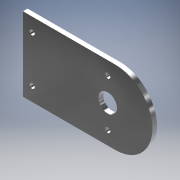
# Autodesk Inventor part: Motor Plate
Saved by Autodesk Inventor 2019.4 (Build 234330000, 330)
## iProperties
Created: 2020-01-22
Part Number: Motor Plate
Material: Aluminum 6061
Document SubType Name: Modeling
Designer: Mark
Mass: 21.6 g
Surface Area: 42 cm^2
Volume: 8 cm^3
Density: 2.7 g/cm^3
Appearance: Aluminum - Flat
Author: Mark
Autodesk Inventor part; units mm, degrees
ref_plane "YZ Plane" through (0, 0, 0) normal (1, 0, 0) x (0, 1, 0)
ref_plane "XZ Plane" through (0, 0, 0) normal (0, 1, 0) x (-1, 0, 0)
ref_plane "XY Plane" through (0, 0, 0) normal (0, 0, 1) x (1, 0, 0)
sketch "Sketch1" plane through (0, 0, 0) normal (0, 0, 1) x (1, 0, 0)
  line L0 (0, 0) -> (20, 0)
  line L1 (20, 0) -> (20, 80)
  line L2 (20, 80) -> (0, 80)
  line L3 (0, 80) -> (0, 0)
  line L4 (20, 0) -> (68, -45) construction
  line L5 (20, 40) -> (120, 40) construction
  line L6 (20, 40) -> (120, 40) construction
  circle A0 centre (94.7172, 40) radius 25.4 construction
  line L7 (94.7172, 40) -> (94.7172, 65.4) construction
  line L8 (94.7172, 40) -> (120.1172, 40) construction
  circle A1 centre (94.7172, 65.4) radius 2.75
  circle A2 centre (94.7172, 14.6) radius 2.75
  line L9 (20, 80) -> (140, 80)
  line L10 (140, 80) -> (140, 0)
  line L11 (140, 0) -> (20, 0)
  line L12 (20, 0) -> (20, 80)
  circle A3 centre (94.7172, 40) radius 10
  line L13 (68, -45) -> (94.7172, 40) construction
  circle A4 centre (94.7172, 40) radius 2.5 construction
  dimension "d0" = 20
  dimension "d1" = 80
  dimension "d15" = 45
  dimension "d16" = 48
  dimension "d17" = 100
  dimension "d18" = 0
  dimension "d20" = 50.8
  dimension "d21" = 90
  dimension "d22" = 5.5
  dimension "d23" = 5.5
  dimension "d24" = 120
  dimension "d25" = 80
  dimension "d26" = 20
  dimension "d29" = 89.1
  dimension "d30" = 5
  constraints: 28 end point, 5 centre point, 5 horizontal, 4 parallel, 3 coincident, 3 point on line, 2 equal length, 2 perpendicular, 2 point on circle, 1 concentric, 1 midpoint
  measures "d0" distance of L2.end L1.end
  measures "d1" distance of L1.end L0.end
  measures "d15" vertical distance of L0.end L4.end
  measures "d16" horizontal distance of L4.end L0.end
  measures "d17" distance of L5.start L5.end
  measures "d18" distance between parallel lines of L5 L6
  measures "d20" diameter of A0
  measures "d21" angle of L8 L7
  measures "d22" diameter of A1
  measures "d23" diameter of A2
  measures "d24" distance of L10.end L11.end
  measures "d25" distance of L9.end L10.end
  measures "d26" diameter of A3
  measures "d29" distance of L4.end L13.end
  measures "d30" diameter of A4
extrude "Extrusion1" add sketch "Sketch1" along normal blind 5
sketch "Sketch2" plane through (0, 0, 5) normal (0, 0, 1) x (1, 0, 0)
  circle A0 centre (10, 15) radius 2.75
  circle A1 centre (10, 65) radius 2.75
  line L0 (0, 80) -> (0, 0) projected
  line L1 (140, 80) -> (0, 80) projected
  line L2 (0, 0) -> (140, 0) projected
  line L3 (20, 0) -> (20, 80)
  dimension "d7" = 5.5
  dimension "d8" = 5.5
  dimension "d9" = 10
  dimension "d10" = 15
  dimension "d11" = 15
  dimension "d12" = 10
  dimension "d27" = 20
  constraints: 2 centre point, 2 end point
  measures "d7" diameter of A0
  measures "d8" diameter of A1
  measures "d9" distance from line of L0 A1.centre
  measures "d10" distance from line of A1.centre L1
  measures "d11" distance from line of L2 A0.centre
  measures "d12" distance from line of L3 A0.centre
  measures "d27" distance between parallel lines of L0 L3
extrude "Extrusion2" cut sketch "Sketch2" against normal blind 5 contours A0 | A1
fillet "Fillet1" radius 40 2 edges at (140, 80, 2.5) (140, 0, 2.5)
body "Solid1"
